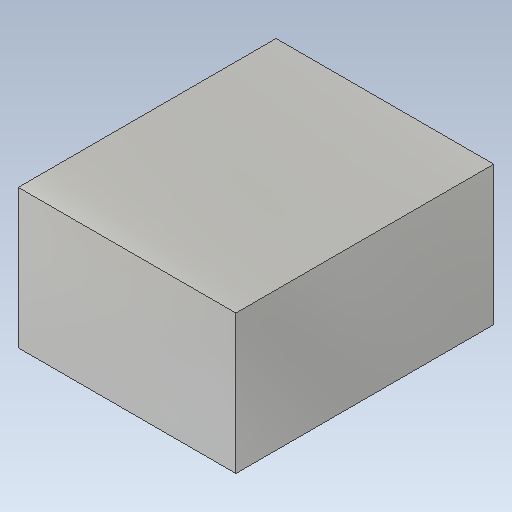
# Autodesk Inventor part: housing
Saved by Autodesk Inventor 2020 (Build 240168000, 168)
## iProperties
Created: 2017-11-24
Part Number: housing
Material: Generic
Document SubType Name: Modeling
Designer: stedrock
Density: 1 g/cm^3
Appearance: Default
Mass: 1661.66 g
Surface Area: 871.84 cm^2
Volume: 1661.66 cm^3
Author: stedrock
Autodesk Inventor part; units mm, degrees
ref_plane "YZ Plane" through (0, 0, 0) normal (1, 0, 0) x (0, 1, 0)
ref_plane "XZ Plane" through (0, 0, 0) normal (0, 1, 0) x (-1, 0, 0)
ref_plane "XY Plane" through (0, 0, 0) normal (0, 0, 1) x (1, 0, 0)
sketch "Sketch1" plane through (0, 0, 0) normal (0, 1, 0) x (-1, 0, 0)
  line L0 (-65, 77) -> (65, 77)
  line L1 (65, 77) -> (65, -77)
  line L2 (65, -77) -> (-65, -77)
  line L3 (-65, -77) -> (-65, 77)
  line L4 (-65, 77) -> (65, -77) construction
  line L5 (65, 77) -> (-65, -77) construction
  point P0 (0, 0)
  dimension "d0" = 130
  dimension "d1" = 154
  constraints: 12 end point, 2 midpoint, 2 parallel, 1 horizontal, 1 perpendicular
  measures "d0" distance of L1.end L2.end
  measures "d1" distance of L0.end L1.end
extrude "Extrusion1" add sketch "Sketch1" along normal blind 83
body "Solid1"
